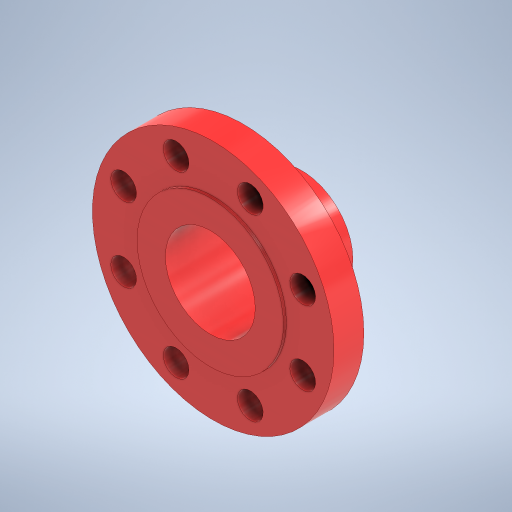
# Autodesk Inventor part: ej_iLogic
Saved by Autodesk Inventor 2023.2 (Build 272271030, 271C)
## iProperties
RuleStatus: InUse
Created: 2023-10-09
Part Number: ej_iLogic
Material: Steel
Document SubType Name: Modeling
Designer: Cris Pat
Density: 7.85 g/cm^3
Appearance: Light Red
Mass: 4847.3 g
Surface Area: 925.18 cm^2
Volume: 617.49 cm^3
Author: Cris Pat
Autodesk Inventor part; units mm, degrees
ref_plane "YZ Plane" through (0, 0, 0) normal (1, 0, 0) x (0, 1, 0)
ref_plane "XZ Plane" through (0, 0, 0) normal (0, 1, 0) x (-1, 0, 0)
ref_plane "XY Plane" through (0, 0, 0) normal (0, 0, 1) x (1, 0, 0)
sketch "Sketch1" plane through (0, 0, 0) normal (0, 0, 1) x (1, 0, 0)
  circle A0 centre (0, 0) radius 104.775
  dimension "d_externo" = 209.55
  constraints: 1 centre point, 1 coincident
  measures "d_externo" diameter of A0
extrude "Diametro externo" add sketch "Sketch1" against normal blind 28.448
sketch "Sketch2" plane through (0, 0, 0) normal (0, 0, 1) x (1, 0, 0)
  circle A0 centre (0, 0) radius 104.775 projected
  circle A1 centre (0, 0) radius 63.5
  dimension "d_resaltado" = 127
  constraints: 1 centre point, 1 coincident
  measures "d_resaltado" diameter of A1
extrude "Resaltado" cut sketch "Sketch2" against normal blind 2.5
sketch "Sketch3" plane through (0, 0, 0) normal (0, 1, 0) x (-1, 0, 0)
  line L0 (-104.775, -28.448) -> (104.775, -28.448) construction
  line L1 (63.5, 0) -> (-63.5, 0) construction
  line L2 (0, -83.82) -> (0, 13.97) projected
  line L3 (0, -28.448) -> (0, -79.248)
  line L4 (0, -79.248) -> (44.45, -79.248)
  line L5 (44.45, -79.248) -> (44.45, -66.548)
  line L6 (44.45, -66.548) -> (58.674, -28.448)
  line L7 (58.674, -28.448) -> (0, -28.448)
  point P0 (0, 0)
  point P1 (0, -28.448)
  point P2 (0, -79.248)
  dimension "dia_a" = 88.9
  dimension "dia_m" = 117.348
  dimension "d8" = 12.7
  dimension "altura_h" = 79.248
  constraints: 10 end point, 2 collinear, 2 perpendicular
  measures "dia_a" diameter of L5 L2
  measures "dia_m" diameter of L6.end L2
  measures "d8" distance from line of L5.end L4
  measures "altura_h" distance between parallel lines of L1 L4
revolve "Cuello" add sketch "Sketch3" angle 360 about axis through (0, 0, -10) along (0, 0, 1)
sketch "Sketch4" plane through (0, 0, 0) normal (0, 0, 1) x (1, 0, 0)
  circle A0 centre (0, 0) radius 38.989
  dimension "d_interior" = 77.978
  constraints: 1 centre point, 1 coincident
  measures "d_interior" diameter of A0
extrude "Diametro interior" cut sketch "Sketch4" against normal through all
sketch "Sketch5" plane through (0, 0, 0) normal (0, 0, 1) x (1, 0, 0)
  line L0 (0, -106.68) -> (0, 106.68) construction
  circle A0 centre (0, 0) radius 84.074 construction
  line L1 (0, 0) -> (32.1737, 77.6742) construction
  dimension "BCD" = 168.148
  dimension "ang_a1" = 22.5
  constraints: 2 coincident, 2 end point, 3 other
  measures "ang_a1" angle of L0 L1
hole "Agujero union" at (32.1737, 77.6742, 0) direction (0, 0, -1) diameter 22.352 end through all
pattern_circular "Patron agujero" count 8 over 360 about axis through (0, 0, -10) along (0, 0, 1) of "Agujero union"
sketch3d "Sketch6"
  constraints: 2 centre point, 2 coincident, 1 concentric, 1 other
feature "RANURA_ORING:1" [suppressed]
equation "\"d8\" = -0.25 * espesor + 0.25 * altura_h"
equation "\"espesor\" = 28.448"
body "Solid1"
